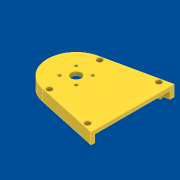
# Autodesk Inventor part: J1-sketch
Saved by Autodesk Inventor 2018 (Build 220112000, 112)
## iProperties
Created: 2019-11-26
Part Number: J1-sketch
Material: Generic
Document SubType Name: Modeling
Designer: Bunny320
Density: 1 g/cm^3
Appearance: Glossy - Gold
Author: Bunny320
## iProperties of the stored document 102-top-motor_3DPrint.ipt
Created: 2019-11-29
Part Number: 102-top-motor_3DPrint
Material: Generic
Document SubType Name: Modeling
Designer: mo
Density: 1 g/cm^3
Appearance: Default
Author: mo
Autodesk Inventor part; units mm, degrees
ref_plane "YZ Plane" through (0, 0, 0) normal (1, 0, 0) x (0, 1, 0)
ref_plane "XZ Plane" through (0, 0, 0) normal (0, 1, 0) x (-1, 0, 0)
ref_plane "XY Plane" through (0, 0, 0) normal (0, 0, 1) x (1, 0, 0)
sketch "Sketch1" plane through (0, 0, 0) normal (0, 0, 1) x (1, 0, 0)
  circle A0 centre (0, 0) radius 30.5
  circle A1 centre (141.8, 0) radius 60.5
  line L0 (129.0003, 59.1305) -> (-6.4528, 29.8096)
  line L1 (-6.4528, -29.8096) -> (129.0003, -59.1305)
  line L2 (60, 44.1943) -> (60, -44.1943)
  dimension "d0" = 61
  dimension "d1" = 121
  dimension "d2" = 141.8
  dimension "d3" = 60
  constraints: 6 end point, 4 point on circle, 4 tangent, 2 centre point, 2 point on line, 1 coincident, 1 horizontal alignment, 1 vertical
  measures "d0" diameter of A0
  measures "d1" diameter of A1
  measures "d2" distance of A1.centre point (0, 0)
  measures "d3" distance from line of point (0, 0) L2
extrude "Extrusion1" add sketch "Sketch1" against normal blind 12 contours A0 | A0 L0 L2 L1
shell "Shell1" thickness 4 removed faces 1 at (37.8491, -9.9365, -12)
sketch "Sketch6" plane through (0, 0, 0) normal (0, 0, 1) x (1, 0, 0)
  point P0 (0, 0)
  point P1 (0, 0)
  constraints: 1 coincident
hole "Hole3" at (0, 0, 0) direction (0, 0, -1) diameter 11 end through all
sketch "Sketch5" plane through (56, -39.2358, -4) normal (0, 0, -1) x (-1, 0, 0)
  line L0 (64.8388, 48.0747) -> (47.1612, 48.0747)
  line L1 (47.1612, 48.0747) -> (47.1612, 30.397)
  line L2 (47.1612, 30.397) -> (64.8388, 30.397)
  line L3 (64.8388, 30.397) -> (64.8388, 48.0747)
  line L4 (64.8388, 48.0747) -> (47.1612, 30.397) construction
  line L5 (47.1612, 48.0747) -> (64.8388, 30.397) construction
  point P0 (56, 39.2358)
  dimension "d16" = 25
  constraints: 12 end point, 4 coincident, 2 midpoint, 2 parallel, 2 perpendicular, 1 horizontal
  measures "d16" distance of L0.start L1.end
hole "Hole2" at (8.8388, -8.8388, -4) at (-8.8388, -8.8388, -4) at (-8.8388, 8.8388, -4) at (8.8388, 8.8388, -4) direction (0, 0, 1) diameter 3.4 end through all countersink diameter 6.3 countersink angle 90 clearance for "Countersunk Flat Head Screw ISO 2009/7046" size "M3" standard "ISO"
sketch "Sketch7" plane through (56, -39.2358, -4) normal (0, 0, -1) x (-1, 0, 0)
  line L0 (26.9325, 5.83) -> (-25.6804, -5.5589)
  line L1 (-25.6804, -5.5589) -> (-25.6804, 84.0306)
  line L2 (-25.6804, 84.0306) -> (28.864, 72.2236)
  line L3 (28.864, 72.2236) -> (24.7276, 5.3527)
  line L4 (61.6065, 13.3357) -> (0, 0) projected
  line L5 (0, 78.4716) -> (61.6065, 65.136) projected
  point P0 (56, 39.2358)
  constraints: 8 end point, 2 collinear, 1 point on line, 1 vertical
extrude "Extrusion2" cut sketch "Sketch7" along normal through all
sketch "Sketch8" plane through (-5.6065, 25.9001, -12) normal (0.2115656, -0.9773638, 0) x (0.9773638, 0.2115656, 0)
  line L0 (0, 8) -> (0, 0) projected
  line L1 (67.126, 0) -> (0, 0) projected
  line L2 (0, 8) -> (8, 8)
  line L3 (8, 8) -> (8, 0)
  line L4 (8, 0) -> (0, 0)
  line L5 (0, 0) -> (0, 8)
  line L6 (53, 8) -> (61, 8)
  line L7 (61, 8) -> (61, 0)
  line L8 (61, 0) -> (53, 0)
  line L9 (53, 0) -> (53, 8)
  point P0 (0, 12)
  dimension "d33" = 8
  dimension "d34" = 8
  dimension "d35" = 45
  constraints: 16 end point, 4 parallel, 3 point on line, 2 horizontal, 2 perpendicular
  measures "d33" distance between parallel lines of L3 L0
  measures "d34" distance between parallel lines of L7 L9
  measures "d35" distance between parallel lines of L9 L3
extrude "Extrusion3" add sketch "Sketch8" along normal blind 4
sketch "Sketch9" plane through (0, 0, -12) normal (0, 0, -1) x (-1, 0, 0)
  line L0 (4.7602, 21.9907) -> (-3.0587, 23.6832) projected
  line L1 (-60, 44.1943) -> (6.4528, 29.8096) projected
  line L2 (-46.1938, 37.1131) -> (-47.0401, 33.2037) projected
  line L3 (-47.0401, 33.2037) -> (-53.1727, 42.6863)
  line L4 (-1.3662, 31.5021) -> (4.7602, 21.9907)
  line L5 (-3.0587, 23.6832) -> (6.4528, 29.8096)
  line L6 (-47.0401, 33.2037) -> (-54.859, 34.8962) projected
  line L7 (-54.859, 34.8962) -> (-45.3475, 41.0226)
  point P0 (0, 0)
  point P1 (-50.1032, 37.9594)
  point P2 (1.697, 26.7464)
  constraints: 8 end point, 2 midpoint, 2 point on line
hole "Hole4" at (50.1032, 37.9594, -12) at (-1.697, 26.7464, -12) direction (0, 0, 1) diameter 3.4 end through all clearance for "Countersunk Flat Head Screw ISO 2009/7046" size "M3" standard "ISO"
sketch "Sketch10" plane through (0, 0, 0) normal (0, 0, 1) x (1, 0, 0)
  circle A0 centre (50.1032, 37.9594) radius 1.7 projected
  circle A1 centre (-1.697, 26.7464) radius 1.7 projected
  point P0 (0, 0)
  constraints: 2 coincident
hole "Hole5" at (50.1032, 37.9594, 0) at (-1.697, 26.7464, 0) direction (0, 0, -1) diameter 6 depth 8
mirror "Mirror1" about plane through (0, 0, 0) normal (0, 1, 0) of "Extrusion3", "Hole4", "Hole5"
equation "\"d34\" = d33"
body "Solid1"
